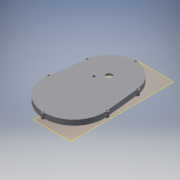
# Autodesk Inventor part: case part 2
Saved by Autodesk Inventor 2017 (Build 210142000, 142)
## iProperties
Created: 2018-04-17
Part Number: case part 2
Material: Generic
Document SubType Name: Modeling
Designer: RKL
Density: 1 g/cm^3
Appearance: Default
Author: RKL
Autodesk Inventor part; units mm, degrees
ref_plane "YZ Plane" through (0, 0, 0) normal (1, 0, 0) x (0, 1, 0)
ref_plane "XZ Plane" through (0, 0, 0) normal (0, 1, 0) x (-1, 0, 0)
ref_plane "XY Plane" through (0, 0, 0) normal (0, 0, 1) x (1, 0, 0)
ref_plane "Work Plane1" through (0, 0, 0) normal (0, 0, 1) x (1, 0, 0)
sketch "Sketch1" plane through (0, 0, 0) normal (0, 0, 1) x (1, 0, 0)
  circle A0 centre (-101.7655, -13.9736) radius 1.397 construction
  circle A1 centre (-129.7655, 19.0264) radius 1.397 construction
  circle A2 centre (-129.7655, -13.9736) radius 1.397 construction
  circle A3 centre (-101.7655, 19.0264) radius 1.397 construction
  circle A4 centre (-43.6844, 106.2389) radius 2.159 projected
  circle A5 centre (-48.0429, -103.7159) radius 2.159 projected
  circle A6 centre (14.7425, 52.5147) radius 2.159 projected
  circle A7 centre (-104.2906, 54.9857) radius 2.159 projected
  arc A8 (-39.1921, 105.9768) -> (-48.1838, 106.1635) centre (-43.6844, 106.2389) ccw projected
  arc A9 (-48.1838, 106.1635) -> (-103.4691, 59.4101) centre (-44.9297, 46.2518) ccw projected
  arc A10 (-103.4691, 59.4101) -> (-104.9457, 50.5336) centre (-104.2906, 54.9857) ccw projected
  line L0 (-104.9457, 50.5336) -> (-109.0664, 22.5264) projected
  line L1 (-133.7655, 22.5264) -> (-109.0664, 22.5264) construction
  line L2 (-133.7655, -17.4736) -> (-133.7655, 22.5264) construction
  line L3 (-133.7655, -17.4736) -> (-119.9083, -25.4741) construction
  arc A11 (-119.9083, -25.4741) -> (-116.3561, -28.0122) centre (-115.8445, -23.5414) ccw projected
  arc A12 (-116.3561, -28.0122) -> (-52.5366, -103.4779) centre (-46.5901, -33.731) ccw projected
  arc A13 (-52.5366, -103.4779) -> (-43.5432, -103.6646) centre (-48.0429, -103.7159) ccw projected
  arc A14 (-43.5432, -103.6646) -> (23.3532, -30.9125) centre (-46.5901, -33.731) ccw projected
  arc A15 (23.3532, -30.9125) -> (22.5578, -21.9488) centre (23.0275, -26.4243) ccw projected
  line L4 (22.5578, -21.9488) -> (15.2122, 48.0393) projected
  arc A16 (15.2122, 48.0393) -> (14.1053, 56.9693) centre (14.7425, 52.5147) ccw projected
  arc A17 (14.1053, 56.9693) -> (-39.1921, 105.9768) centre (-44.9297, 46.2518) ccw projected
  circle A18 centre (-115.8445, -23.5414) radius 2.159 projected
  circle A19 centre (23.0275, -26.4243) radius 2.159 projected
  circle A20 centre (-44.9297, 46.2518) radius 17.5 projected
  circle A21 centre (-46.5901, -33.731) radius 17.5 projected
  circle A22 centre (-112.6295, 11.4221) radius 4 construction
  circle A23 centre (-121.7655, -6.3693) radius 4 construction
  arc A24 (-115.1894, -19.0893) -> (-119.9083, -25.4741) centre (-115.8445, -23.5414) ccw
  line L5 (-109.0664, 22.5264) -> (-115.1894, -19.0893)
  point P0 (0, 0)
  constraints: 2 end point, 2 point on circle, 1 centre point, 1 coincident, 1 collinear
extrude "Extrusion1" add sketch "Sketch1" along normal blind 10
sketch "Sketch2" plane through (0, 0, 10) normal (0, 0, 1) x (1, 0, 0)
  circle A0 centre (-112.6295, 11.4221) radius 4 projected
  point P0 (0, 0)
extrude "Extrusion2" cut sketch "Sketch2" against normal through all
sketch "Sketch3" plane through (0, 0, 10) normal (0, 0, 1) x (1, 0, 0)
  arc A0 (-111.2528, 7.6664) -> (-110.2294, 14.622) centre (-112.6295, 11.4221) ccw projected
  line L0 (-111.2528, 7.6664) -> (-115.1894, -19.0893) projected
  arc A1 (-115.1894, -19.0893) -> (-116.3561, -28.0122) centre (-115.8445, -23.5414) ccw projected
  arc A2 (-116.3561, -28.0122) -> (-52.5366, -103.4779) centre (-46.5901, -33.731) ccw projected
  arc A3 (-52.5366, -103.4779) -> (-43.5432, -103.6646) centre (-48.0429, -103.7159) ccw projected
  arc A4 (-43.5432, -103.6646) -> (23.3532, -30.9125) centre (-46.5901, -33.731) ccw projected
  arc A5 (23.3532, -30.9125) -> (22.5578, -21.9488) centre (23.0275, -26.4243) ccw projected
  line L1 (22.5578, -21.9488) -> (15.2122, 48.0393) projected
  arc A6 (15.2122, 48.0393) -> (14.1053, 56.9693) centre (14.7425, 52.5147) ccw projected
  arc A7 (14.1053, 56.9693) -> (-39.1921, 105.9768) centre (-44.9297, 46.2518) ccw projected
  arc A8 (-39.1921, 105.9768) -> (-48.1838, 106.1635) centre (-43.6844, 106.2389) ccw projected
  arc A9 (-48.1838, 106.1635) -> (-103.4691, 59.4101) centre (-44.9297, 46.2518) ccw projected
  arc A10 (-103.4691, 59.4101) -> (-104.9457, 50.5336) centre (-104.2906, 54.9857) ccw projected
  line L2 (-104.9457, 50.5336) -> (-110.2294, 14.622) projected
  circle A11 centre (-43.6844, 106.2389) radius 2.159 projected
  circle A12 centre (-48.0429, -103.7159) radius 2.159 projected
  circle A13 centre (14.7425, 52.5147) radius 2.159 projected
  circle A14 centre (-104.2906, 54.9857) radius 2.159 projected
  circle A15 centre (-115.8445, -23.5414) radius 2.159 projected
  circle A16 centre (23.0275, -26.4243) radius 2.159 projected
  circle A17 centre (-44.9297, 46.2518) radius 17.5 projected
  circle A18 centre (-46.5901, -33.731) radius 17.5 projected
  circle A19 centre (-46.5901, -33.731) radius 7
  circle A20 centre (-44.9297, 46.2518) radius 7
  point P0 (0, 0)
  dimension "d4" = 14
  constraints: 2 centre point, 2 coincident, 1 equal radius
  measures "d4" diameter of A19
extrude "Extrusion3" add sketch "Sketch3" along normal blind 2 contours A0 L2 A10 A9 A8 A7 A6 L1 A5 A4 A3 A2 A1 L0 | A17 | A18 | A19
sketch "Sketch4" plane through (0, 0, 12) normal (0, 0, 1) x (1, 0, 0)
  circle A0 centre (-61.4531, 27.4907) radius 3 projected
  point P0 (0, 0)
extrude "Extrusion4" cut sketch "Sketch4" against normal through all
body "Solid1"
